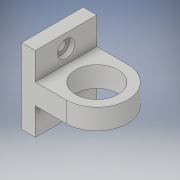
# Autodesk Inventor part: Organic Filter Holder
Saved by Autodesk Inventor 2019 (Build 230136000, 136)
## iProperties
Created: 2019-08-20
Part Number: Organic Filter Holder
Material: Generic
Document SubType Name: Modeling
Designer: dewanlab
Density: 1 g/cm^3
Appearance: Default
Author: dewanlab
Autodesk Inventor part; units mm, degrees
ref_plane "YZ Plane" through (0, 0, 0) normal (1, 0, 0) x (0, 1, 0)
ref_plane "XZ Plane" through (0, 0, 0) normal (0, 1, 0) x (-1, 0, 0)
ref_plane "XY Plane" through (0, 0, 0) normal (0, 0, 1) x (1, 0, 0)
sketch "Sketch1" plane through (0, 0, 0) normal (1, 0, 0) x (0, 1, 0)
  line L0 (33.4134, 34.8656) -> (-36.4366, 34.8656)
  line L1 (-36.4366, 34.8656) -> (-36.4366, -22.2844)
  line L2 (-36.4366, -22.2844) -> (33.4134, -22.2844)
  line L3 (33.4134, -22.2844) -> (33.4134, 34.8656)
  point P0 (0, 0)
  dimension "d0" = 57.15
  dimension "d1" = 69.85
  constraints: 8 end point, 2 parallel, 1 horizontal, 1 perpendicular
  measures "d0" distance between parallel lines of L2 L0
  measures "d1" distance between parallel lines of L1 L3
extrude "Extrusion1" add sketch "Sketch1" along normal blind 12.7
sketch "Sketch2" plane through (12.7, 0, 0) normal (1, 0, 0) x (0, 0, -1)
  line L0 (-34.8656, 8.0134) -> (22.2844, 8.0134)
  line L1 (22.2844, 8.0134) -> (22.2844, -11.0366)
  line L2 (22.2844, -11.0366) -> (-34.8656, -11.0366)
  line L3 (-34.8656, -11.0366) -> (-34.8656, 8.0134)
  line L4 (22.2844, -36.4366) -> (22.2844, 33.4134) projected
  line L5 (-34.8656, 33.4134) -> (-34.8656, -36.4366) projected
  line L6 (22.2844, 33.4134) -> (-34.8656, 33.4134) projected
  point P0 (0, 0)
  dimension "d5" = 0
  dimension "d9" = 57.15
  dimension "d16" = 19.05
  dimension "d17" = 25.4
  constraints: 8 end point, 2 parallel, 1 horizontal, 1 perpendicular
  measures "d5" distance between parallel lines of L5 L3
  measures "d9" distance between parallel lines of L1 L3
  measures "d16" distance between parallel lines of L2 L0
  measures "d17" distance between parallel lines of L0 L6
extrude "Extrusion2" add sketch "Sketch2" along normal blind 57.15 contours L0 L1 L2 L3
fillet "Fillet1" radius 28.575 1 edges at (69.85, -1.5116, 34.8656)
fillet "Fillet2" radius 28.575 1 edges at (69.85, -1.5116, -22.2844)
sketch "Sketch3" plane through (12.7, 8.0134, 34.8656) normal (0, 1, 0) x (1, 0, 0)
  circle A0 centre (28.575, 28.575) radius 19.812
  line L0 (0, 0) -> (28.575, 0) projected
  line L1 (0, 57.15) -> (0, 0) projected
  point P0 (-12.7, 34.8656)
  dimension "d11" = 39.624
  dimension "d12" = 28.575
  dimension "d13" = 28.575
  constraints: 1 centre point
  measures "d11" diameter of A0
  measures "d12" distance from line of L0 A0.centre
  measures "d13" distance from line of L1 A0.centre
extrude "Extrusion3" cut sketch "Sketch3" against normal blind 50.8
sketch "Sketch4" plane through (12.7, 0, 0) normal (1, 0, 0) x (0, 0, -1)
  point P0 (0, 0)
sketch "Sketch5" plane through (12.7, 0, 0) normal (1, 0, 0) x (0, 0, -1)
  line L0 (22.2844, -36.4366) -> (22.2844, 33.4134) projected
  line L1 (22.2844, 33.4134) -> (-34.8656, 33.4134) projected
  point P0 (0, 0)
  point P1 (-6.2906, 20.7134)
  dimension "d25" = 28.575
  dimension "d35" = 12.7
  measures "d25" distance from line of L0 point (-6.291, 20.713)
  measures "d35" distance from line of L1 point (-6.291, 20.713)
hole "Hole1" at (12.7, 20.7134, 6.2906) direction (-1, 0, 0) diameter 8.4328 end through all counterbore diameter 15.875 counterbore depth 4.7625 clearance for "Socket Head Cap Screw" size "5/16" standard "Ansi Unified Screw Threads"
sketch "Sketch6" plane through (12.7, 0, 0) normal (1, 0, 0) x (0, 0, -1)
  line L0 (22.2844, -36.4366) -> (22.2844, 33.4134) projected
  line L1 (-34.8656, -36.4366) -> (22.2844, -36.4366) projected
  point P0 (0, 0)
  point P1 (-6.2906, -23.7366)
  dimension "d33" = 28.575
  dimension "d34" = 12.7
  measures "d33" distance from line of L0 point (-6.291, -23.737)
  measures "d34" distance from line of L1 point (-6.291, -23.737)
hole "Hole2" at (12.7, -23.7366, 6.2906) direction (-1, 0, 0) diameter 8.4328 end through all counterbore diameter 15.875 counterbore depth 4.7625 clearance for "Socket Head Cap Screw" size "5/16" standard "Ansi Unified Screw Threads"
body "Solid1"
